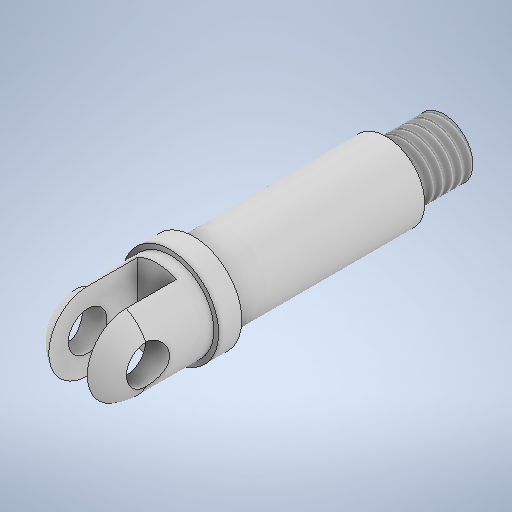
# Autodesk Inventor part: 13
Saved by Autodesk Inventor 2025.1 (Build 291241000, 241)
## iProperties
Created: 2024-09-13
Part Number: 13
Material: Generisch
Document SubType Name: Modeling
Designer: ffogue
Density: 1 g/cm^3
Appearance: Vorgabe
Author: ffogue
Autodesk Inventor part; units mm, degrees
ref_plane "XZ Plane" through (0, 0, 0) normal (0, 1, 0) x (-1, 0, 0)
sketch "Sketch1" plane through (0, 0, 0) normal (1, 0, 0) x (0, 1, 0)
  arc A0 (4.5, 4.5) -> (0, 0) centre (4.5, 0) ccw
  line L0 (4.5, 4.5) -> (11.1, 4.5)
  line L1 (13.5, 4) -> (33.5, 4)
  line L2 (33.5, 4) -> (33.5, 3)
  line L3 (31.6452, 0) -> (4.5, 0)
  line L4 (33.5, 3) -> (39.5, 3)
  line L5 (39.5, 3) -> (39.5, 0)
  line L6 (39.5, 0) -> (31.6452, 0)
  line L7 (11.1, 4.5) -> (11.1, 5)
  line L8 (11.1, 5) -> (13.5, 5)
  line L9 (13.5, 5) -> (13.5, 4)
  line L10 (4.5, 0) -> (0, 0)
  point P0 (0, 0)
  dimension "d0" = 4.5
  dimension "d5" = 8
  dimension "d6" = 20
  dimension "d7" = 6
  dimension "d8" = 6
  dimension "d10" = 10
  dimension "d11" = 35
  dimension "d12" = 6.6
  constraints: 22 end point, 5 horizontal, 4 perpendicular, 2 coincident, 2 point on circle, 1 centre point, 1 horizontal alignment, 1 point on line, 1 tangent, 1 vertical
  measures "d0" radius of A0
  measures "d5" diameter of L1 L3
  measures "d6" distance of L1.start L1.end
  measures "d7" distance of L2.end L4.end
  measures "d8" diameter of L4 L6
  measures "d10" diameter of L8 L3
  measures "d11" distance from line of A0.centre L5
  measures "d12" distance from line of A0.centre L7
revolve "Revolution1" add sketch "Sketch1" angle 360 about axis through (0, 31.6452, 0) along (0, -1, 0)
ref_plane "Work Plane4" through (0, 0, 0) normal (0, 0, 1) x (1, 0, 0)
sketch "Sketch2" plane through (0, 0, 0) normal (0, 0, 1) x (1, 0, 0)
  line L0 (-2, 9.7) -> (2, 9.7)
  line L1 (2, 9.7) -> (2, 0.4689)
  arc A0 (-4.5, 4.5) -> (4.5, 4.5) centre (0, 4.5) ccw projected
  line L2 (-2, 9.7) -> (-2, 0.4689)
  arc A1 (-2, 0.4689) -> (2, 0.4689) centre (0, 4.5) ccw
  point P0 (0, 0)
  point P1 (0, 0)
  dimension "d18" = 4
  dimension "d19" = 2
  dimension "d20" = 9.7
  constraints: 7 point on circle, 6 end point, 1 centre point, 1 concentric, 1 horizontal, 1 parallel, 1 perpendicular
  measures "d18" distance of L0.start L0.end
  measures "d19" distance from line of L1 A0.centre
  measures "d20" distance from line of point (0, 0) L0
extrude "Extrusion1" cut sketch "Sketch2" along normal through all both and the other way through all
ref_plane "Work Plane5" through (4.5, 0, 0) normal (1, 0, 0) x (0, 1, 0)
sketch "Sketch3" plane through (4.5, 0, 0) normal (1, 0, 0) x (0, 1, 0)
  line L0 (4.5, 4.0311) -> (4.5, -4.0311) projected
  line L1 (4.5, 4.0311) -> (4.5, -4.0311) projected
  point P0 (0, 0)
  point P1 (4.5, 0)
  point P2 (4.5, 0)
  constraints: 2 midpoint, 1 horizontal alignment
hole "Hole1" at (4.5, 4.5, 0) direction (-1, 0, 0) diameter 4 end through all
thread "Thread1" size "M6x1" class "6g" standard "ISO Metric profile" length 8
equation "\"d19\" = 0.5 * d18"
body "Solid1"
